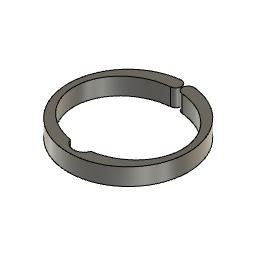
anchor_ring v6 (Autodesk Fusion 360 design; units mm, degrees)
Autodesk Fusion 360 part; units mm, degrees
sketch "Sketch1" plane through (0, 0, 0) normal (0, 0, 1) x (1, 0, 0)
  line L0 (0.1, 8.4995) -> (0.1, 10.4995)
  line L1 (-0.1, 10.4995) -> (-0.1, 8.4995)
  line L2 (-10.5245, 0) -> (10.5245, 0)
  arc A0 (-0.1, 10.4995) -> (0.1, 10.4995) centre (0, 0) ccw
  line L3 (0, 8.6614) -> (0, -8.6614) construction
  ellipse E0 centre (0, 0) end of major axis (9.5, 0) minor radius 8.5
  line L4 (-9.5, 0) -> (9.5, 0)
  line L5 (0, -8.5) -> (0, 8.5)
  dimension "d2" = 21
  dimension "d5" = 0.2
  dimension "d30" = 19
  dimension "d31" = 17
  constraint coincident A0.centre E0.centre
  constraint perpendicular L2 L3
  constraint symmetric L0 L1 L3
  constraint midpoint A0.centre L3
  constraint midpoint A0.centre L2
  constraint coincident E0 L4.start
  constraint coincident E0 L4.end
  constraint coincident E0 L5.start
  constraint coincident E0 L5.end
  constraint perpendicular L3 L4
  constraint coincident L1.end E0
  constraint vertical L1
  constraint coincident L0.start E0
  measures "d2" diameter of A0
  measures "d5" distance of L0 L1
  measures "d30" distance of E0
extrude "Extrude6" add sketch "Sketch1" along normal blind 3 contours L0 L2 A0 E0 | L2 A0 E0 | L1 L2 A0 E0
sketch "Sketch2" plane through (0, 0, 0) normal (0, 1, 0) x (1, 0, 0)
sketch "Sketch3" plane through (0, 0, 2) normal (0, 0, 1) x (-1, 0, 0)
  line L0 (5, 0) -> (-5, 0)
  line L1 (0, -7.3914) -> (0, 7.3914)
  ellipse E0 centre (0, 7.3914) end of major axis (-6, 7.3914) minor radius 3
  line L2 (6, 7.3914) -> (-6.1851, 7.3914)
  line L3 (0, 7.3914) -> (0, 4.3914)
  ellipse E1 centre (0, 7.3914) end of major axis (2, 7.3914) minor radius 2.25
  line L4 (-2, 7.3914) -> (2, 7.3914)
  line L5 (0, 5.1414) -> (0, 9.6414)
  dimension "d15" = 12
  dimension "d16" = 6
  dimension "d17" = 4
  dimension "d18" = 4.5
  constraint horizontal L0
  constraint vertical L1
  constraint midpoint L0 origin
  constraint midpoint L1 origin
  constraint coincident E0 L2.start
  constraint coincident E0 L3.end
  constraint coincident L1 E0.centre
  constraint coincident E1 L4.start
  constraint coincident E1 L4.end
  constraint coincident E1 L5.start
  constraint coincident E1 L5.end
  constraint concentric E0 E1
  constraint collinear L2 L4
  constraint coincident L1.end E0.centre
  measures "d15" distance of E0
  measures "d16" distance of E0
  measures "d17" distance of E1
extrude "Extrude7" cut sketch "Sketch3" along normal up to surface (-2 mm away) and the other way up to surface (-1 mm away) contours L1 L2 L3 E1 L4 L5 | L1 L2 L3 E1 L4 L5 | L2 E1 L4 L5 | L2 E1 L4 L5
fillet "Fillet1" radius 1 4 edges at (-0.1, 8.4995, 1.5) (-0.1, 10.4995, 1.5) (0.1, 8.4995, 1.5) (0.1, 10.4995, 1.5)
extrude "Extrude2" [suppressed]
extrude "Extrude3" [suppressed]
extrude "Extrude4" [suppressed]
extrude "Extrude5" [suppressed]
